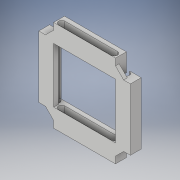
# Autodesk Inventor part: 20_Rect_Aperture_Insert_half
Saved by Autodesk Inventor 2019 (Build 230136000, 136)
## iProperties
Created: 2020-03-02
Part Number: 20_Rect_Aperture_Insert_half
Material: Generic
Document SubType Name: Modeling
Designer: marsikovabarbora
Density: 1 g/cm^3
Appearance: Default
Author: marsikovabarbora
Autodesk Inventor part; units mm, degrees
ref_plane "YZ Plane" through (0, 0, 0) normal (1, 0, 0) x (0, 1, 0)
ref_plane "XZ Plane" through (0, 0, 0) normal (0, 1, 0) x (-1, 0, 0)
ref_plane "XY Plane" through (0, 0, 0) normal (0, 0, 1) x (1, 0, 0)
sketch "Sketch1" plane through (0, 0, 0) normal (0, 0, 1) x (1, 0, 0)
  line L0 (-51.8104, 0) -> (51.8104, 0) construction
  line L1 (0, -35.1144) -> (0, 36.3819) construction
  line L2 (0, 0) -> (26.1682, 26.1682) construction
  line L3 (0, 0) -> (37.0074, 0) construction
  line L4 (16.8, 24.9006) -> (16.8, 21.2406)
  line L5 (16.8, 21.2406) -> (19.0203, 19.0203)
  line L6 (16.8, 24.9006) -> (0, 24.9006)
  line L7 (24.9006, 16.8) -> (21.2406, 16.8)
  line L8 (21.2406, 16.8) -> (19.0203, 19.0203)
  line L9 (24.9006, 16.8) -> (24.9006, 0)
  line L10 (0, 0) -> (-37.0074, 0) construction
  line L11 (-16.8, 24.9006) -> (-16.8, 21.2406)
  line L12 (-16.8, 21.2406) -> (-19.0203, 19.0203)
  line L13 (-16.8, 24.9006) -> (0, 24.9006)
  line L14 (-24.9006, 16.8) -> (-24.9006, 0)
  line L15 (-24.9006, 16.8) -> (-21.2406, 16.8)
  line L16 (-21.2406, 16.8) -> (-19.0203, 19.0203)
  line L17 (16.8, -24.9006) -> (16.8, -21.2406)
  line L18 (16.8, -21.2406) -> (19.0203, -19.0203)
  line L19 (16.8, -24.9006) -> (0, -24.9006)
  line L20 (24.9006, -16.8) -> (24.9006, 0)
  line L21 (24.9006, -16.8) -> (21.2406, -16.8)
  line L22 (21.2406, -16.8) -> (19.0203, -19.0203)
  line L23 (-16.8, -24.9006) -> (-16.8, -21.2406)
  line L24 (-16.8, -21.2406) -> (-19.0203, -19.0203)
  line L25 (-16.8, -24.9006) -> (0, -24.9006)
  line L26 (-24.9006, -16.8) -> (-24.9006, 0)
  line L27 (-24.9006, -16.8) -> (-21.2406, -16.8)
  line L28 (-21.2406, -16.8) -> (-19.0203, -19.0203)
  line L29 (-16.8, -16.8) -> (16.8, 16.8) construction
  line L30 (17.4242, -17.4242) -> (-16.0391, 16.0391) construction
  line L31 (-16.8, -15) -> (16.8, -15)
  line L32 (16.8, -15) -> (16.8, 15)
  line L33 (16.8, 15) -> (-16.8, 15)
  line L34 (-16.8, 15) -> (-16.8, -15)
  line L35 (-16.8, -15) -> (16.8, 15) construction
  line L36 (16.8, -15) -> (-16.8, 15) construction
  dimension "d0" = 45
  dimension "d1" = 3.14
  dimension "d2" = 3.66
  dimension "d4" = 16.8
  dimension "d16" = 33.6
  dimension "d17" = 30
  constraints: 70 end point, 21 symmetric about line, 4 perpendicular, 4 point on line, 3 midpoint, 2 horizontal, 2 parallel, 1 equal length
  measures "d0" angle of L3 L2
  measures "d1" distance of L4.end L5.end
  measures "d2" distance of L4.start L4.end
  measures "d4" distance of L4.start L6.end
  measures "d16" distance of L32.end L33.end
  measures "d17" distance of L33.end L31.start
extrude "Extrusion1" add sketch "Sketch1" along normal blind 8
sketch "Sketch2" plane through (-16.8, 24.9006, 0) normal (0, 1, 0) x (1, 0, 0)
  line L0 (-8.1006, 0) -> (-4.4406, 0) construction
  line L1 (-8.1006, 0) -> (-8.1006, -8) construction
  line L2 (-4.4406, -8) -> (-8.1006, -8) construction
  line L3 (-4.4406, 0) -> (-4.4406, -8) construction
  line L4 (-4.4406, 0) -> (0, 0) construction
  line L5 (-4.4406, 0) -> (-4.4406, -8) construction
  line L6 (0, -8) -> (-4.4406, -8) construction
  line L7 (0, 0) -> (0, -8) construction
  line L8 (0, 0) -> (33.6, 0) construction
  line L9 (0, 0) -> (0, -8) construction
  line L10 (33.6, -8) -> (0, -8) construction
  line L11 (33.6, 0) -> (33.6, -8) construction
  line L12 (33.6, 0) -> (38.0406, 0) construction
  line L13 (33.6, 0) -> (33.6, -8) construction
  line L14 (38.0406, -8) -> (33.6, -8) construction
  line L15 (38.0406, 0) -> (38.0406, -8) construction
  line L16 (38.0406, 0) -> (41.7006, 0) construction
  line L17 (38.0406, 0) -> (38.0406, -8) construction
  line L18 (41.7006, -8) -> (38.0406, -8) construction
  line L19 (41.7006, 0) -> (41.7006, -8) construction
  line L20 (-0.9933, -0.6346) -> (2.8461, 5.7642) construction
  ellipse E0 centre (4.1754, 7.1215) end of major axis (2.3333, 6.6563) minor radius 1.8997 (5.4585, 5.7204) -> (2.8461, 5.7642) ccw construction
  line L21 (5.4585, 5.7204) -> (9.3415, -1.2728) construction
  line L22 (9.3415, -1.2728) -> (8.4179, -1.2574) construction
  line L23 (8.4179, -1.2574) -> (4.8304, 5.2036) construction
  ellipse E1 centre (5.2675, 5.4463) end of major axis (4.7828, 5.3239) minor radius 0.4999 (4.9945, 5.8651) -> (4.8304, 5.2036) ccw construction
  ellipse E2 centre (4.1754, 7.1215) end of major axis (2.7211, 6.7542) minor radius 1.4998 (4.9945, 5.8651) -> (3.3146, 5.8932) ccw construction
  ellipse E3 centre (3.0277, 5.4838) end of major axis (3.5125, 5.6062) minor radius 0.4999 (3.4564, 5.2266) -> (3.3146, 5.8932) ccw construction
  line L24 (3.4564, 5.2266) -> (-0.3461, -1.1107) construction
  ellipse E4 centre (-1.5262, -2.0366) end of major axis (-0.0719, -1.6693) minor radius 1.4998 (-0.9933, -0.6346) -> (-0.3461, -1.1107) ccw construction
  circle A0 centre (-2.1474, -2.1474) radius 1.7
  line L25 (-4.4406, 0) -> (0, 0) construction
  line L26 (0, 0) -> (-3.5302, -3.5302) construction
  line L27 (0, 0) -> (4.9925, 0) construction
  line L28 (0, 0) -> (2, 0)
  line L29 (0, 0) -> (-1.7777, 0)
  line L30 (-1.7777, 0) -> (-2.227, -0.4493)
  line L31 (0, 0) -> (0, -3.2892)
  line L32 (0, -3.2892) -> (-0.8879, -3.2892)
  point P0 (16.8, 0)
  dimension "d8" = 3.4
  dimension "d9" = 135
  constraints: 16 end point, 3 point on line, 2 point on circle, 1 centre point, 1 equal length, 1 horizontal, 1 parallel, 1 perpendicular, 5 other
  measures "d8" diameter of A0
  measures "d9" angle of L26 L27
extrude "Extrusion2" cut sketch "Sketch2" against normal up to surface (39.9006 mm away)
sketch "Sketch3" plane through (0, 0, 0) normal (0, 0, -1) x (-1, 0, 0)
  line L0 (16.8, 15) -> (16.8, 24.9006) construction
  line L1 (16.8, 24.9006) -> (-16.8, 24.9006) construction
  line L2 (-16.8, 24.9006) -> (-16.8, 21.2406) construction
  line L3 (-16.8, 21.2406) -> (-21.2406, 16.8) construction
  line L4 (-21.2406, 16.8) -> (-24.9006, 16.8) construction
  line L5 (-24.9006, 16.8) -> (-24.9006, -16.8) construction
  line L6 (-24.9006, -16.8) -> (-21.2406, -16.8) construction
  line L7 (-21.2406, -16.8) -> (-16.8, -21.2406) construction
  line L8 (-16.8, -21.2406) -> (-16.8, -24.9006) construction
  line L9 (-16.8, -24.9006) -> (16.8, -24.9006) construction
  line L10 (16.8, -24.9006) -> (16.8, -21.2406) construction
  line L11 (16.8, -21.2406) -> (21.2406, -16.8) construction
  line L12 (21.2406, -16.8) -> (24.9006, -16.8) construction
  line L13 (24.9006, -16.8) -> (24.9006, 16.8) construction
  line L14 (24.9006, 16.8) -> (21.2406, 16.8) construction
  line L15 (21.2406, 16.8) -> (18.5777, 19.4629) construction
  line L16 (21.2406, 16.8) -> (24.9006, 16.8) construction
  line L17 (24.9006, 16.8) -> (21.2406, 16.8) projected
  line L18 (18.5777, 19.4629) -> (18.5777, -15) projected
  line L19 (16.8, 21.2406) -> (21.2406, 16.8) projected
  line L20 (21.2406, 16.8) -> (16.8, 21.2406)
  line L21 (16.8, 21.2406) -> (16.8, 16.8)
  line L22 (16.8, 16.8) -> (21.2406, 16.8)
  line L23 (18.5777, 19.4629) -> (18.5777, -15) projected
  line L24 (18.5777, -15) -> (-16.8, -15) projected
  line L25 (-16.8, -15) -> (-16.8, 15) projected
  line L26 (-16.8, 15) -> (16.8, 15) projected
  point P0 (0, 0)
  point P1 (18.5777, -16.8)
  constraints: 6 end point, 2 collinear, 1 vertical
extrude "Extrusion3" cut sketch "Sketch3" against normal blind 3.9
mirror "Mirror1" about plane through (0, 0, 0) normal (1, 0, 0) of "Extrusion3", "Extrusion2"
sketch "Sketch4" plane through (-16.8, -15, 8) normal (0, 1, 0) x (1, 0, 0)
  line L0 (-1.7777, 8) -> (35.3777, 8) construction
  line L1 (-1.7777, 8) -> (-2.227, 7.5507) construction
  arc A0 (-2.227, 7.5507) -> (-0.8879, 4.7108) centre (-2.1474, 5.8526) ccw construction
  line L2 (-0.8879, 4.7108) -> (0, 4.7108) construction
  line L3 (0, 4.7108) -> (0, 0) construction
  line L4 (33.6, 0) -> (0, 0) construction
  line L5 (33.6, 4.7108) -> (33.6, 0) construction
  line L6 (34.4879, 4.7108) -> (33.6, 4.7108) construction
  arc A1 (34.4879, 4.7108) -> (35.827, 7.5507) centre (35.7474, 5.8526) ccw construction
  line L7 (35.3777, 8) -> (35.827, 7.5507) construction
  circle A2 centre (35.7474, 5.8526) radius 1.7
  circle A3 centre (-2.1474, 5.8526) radius 1.7
  point P0 (16.8, 8)
  constraints: 2 centre point, 2 coincident, 2 concentric
extrude "Extrusion4" cut sketch "Sketch4" against normal blind 10
sketch "Sketch5" plane through (-16.8, 24.9006, 0) normal (0, 1, 0) x (1, 0, 0)
  line L0 (0, 0) -> (33.6, 0) construction
  line L1 (0, 0) -> (0, -8) construction
  line L2 (33.6, -8) -> (0, -8) construction
  line L3 (33.6, 0) -> (33.6, -8) construction
  line L4 (16.8, 0) -> (16.8, -8) construction
  line L5 (33.6, 0) -> (33.6, -8) construction
  line L6 (0, 0) -> (0, -8) construction
  line L7 (33.6, -4) -> (0, -4) construction
  line L8 (2.5, -4) -> (31.1, -4) construction
  line L9 (2.5, -5.75) -> (31.1, -5.75)
  line L10 (31.1, -2.25) -> (2.5, -2.25)
  arc A0 (2.5, -2.25) -> (2.5, -5.75) centre (2.5, -4) ccw
  arc A1 (31.1, -5.75) -> (31.1, -2.25) centre (31.1, -4) ccw
  point P0 (16.8, -4)
  dimension "d20" = 3.5
  dimension "d21" = 2.5
  constraints: 12 end point, 5 midpoint, 4 point on circle, 4 tangent, 2 centre point, 1 parallel, 1 point on line
  measures "d20" distance between parallel lines of L10 L9
  measures "d21" distance from line of L3 L8.end
extrude "Extrusion5" cut sketch "Sketch5" against normal through all
sketch "Sketch6" plane through (0, 0, 8) normal (0, 0, 1) x (1, 0, 0)
  line L0 (-16.8, -15) -> (-16.8, 15) projected
  line L1 (-16.8, 15) -> (16.8, 15) projected
  line L2 (16.8, 15) -> (16.8, -15) projected
  line L3 (16.8, -15) -> (-16.8, -15) projected
  line L4 (16.8, 21.2406) -> (16.8, 24.9006) projected
  line L5 (16.8, 24.9006) -> (-16.8, 24.9006) projected
  line L6 (-16.8, 24.9006) -> (-16.8, 21.2406) projected
  line L7 (-16.8, 21.2406) -> (-21.2406, 16.8) projected
  line L8 (-21.2406, 16.8) -> (-24.9006, 16.8) projected
  line L9 (-24.9006, 16.8) -> (-24.9006, -16.8) projected
  line L10 (-24.9006, -16.8) -> (-21.2406, -16.8) projected
  line L11 (-21.2406, -16.8) -> (-16.8, -21.2406) projected
  line L12 (-16.8, -21.2406) -> (-16.8, -24.9006) projected
  line L13 (-16.8, -24.9006) -> (16.8, -24.9006) projected
  line L14 (16.8, -24.9006) -> (16.8, -21.2406) projected
  line L15 (16.8, -21.2406) -> (21.2406, -16.8) projected
  line L16 (21.2406, -16.8) -> (24.9006, -16.8) projected
  line L17 (24.9006, -16.8) -> (24.9006, 16.8) projected
  line L18 (24.9006, 16.8) -> (21.2406, 16.8) projected
  line L19 (21.2406, 16.8) -> (16.8, 21.2406) projected
  point P0 (0, 0)
extrude "Extrusion6" cut sketch "Sketch6" against normal blind 2.1
body "Solid1"
